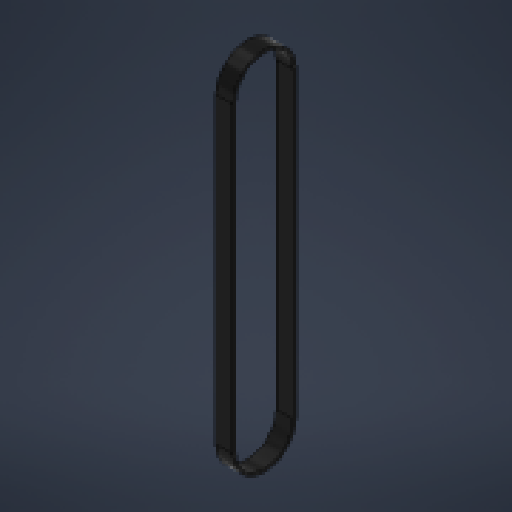
# Autodesk Inventor part: STANDIN,BELT,100T,HTD5mm
Saved by Autodesk Inventor 2026.1 (Build 301233020, 233B)
## iProperties
Created: 2026-02-08
Part Number: STANDIN,BELT,100T,HTD5mm
Material: Nylon 6/6
Document SubType Name: Modeling
Designer: Owen L
Density: 1.13 g/cm^3
Appearance: Smooth - Black
Author: Owen L
Autodesk Inventor part; units mm, degrees
ref_plane "YZ Plane" through (0, 0, 0) normal (1, 0, 0) x (0, 1, 0)
ref_plane "XZ Plane" through (0, 0, 0) normal (0, 1, 0) x (-1, 0, 0)
ref_plane "XY Plane" through (0, 0, 0) normal (0, 0, 1) x (1, 0, 0)
sketch "Sketch1" plane through (0, 0, 0) normal (1, 0, 0) x (0, 1, 0)
  arc A0 (0, -16.7132) -> (0, 16.7132) centre (0, 0) ccw
  arc A1 (-160.4946, 16.7132) -> (-160.4946, -16.7132) centre (-160.4946, 0) ccw
  line L0 (0, 16.7132) -> (-160.4946, 16.7132)
  line L1 (-160.4946, -16.7132) -> (0, -16.7132)
  arc A2 (-160.4946, 15.1257) -> (-160.4946, -15.1257) centre (-160.4946, 0) ccw
  line L2 (-160.4946, -15.1257) -> (0, -15.1257)
  arc A3 (0, -15.1257) -> (0, 15.1257) centre (0, 0) ccw
  line L3 (0, 15.1257) -> (-160.4946, 15.1257)
  dimension "d0" = 16.7132
  dimension "d1" = 160.4946
  dimension "d5" = 1.5875
  constraints: 8 end point, 8 point on circle, 4 centre point, 2 parallel, 2 tangent, 1 coincident, 1 equal radius, 1 horizontal, 1 horizontal alignment, 3 other
  measures "d0" radius of A0
  measures "d1" distance of point (0, 0) A1.centre
  measures "d5" distance between parallel lines of L0 L3
extrude "Extrusion1" add sketch "Sketch1" along normal blind 9
body "Solid1"
